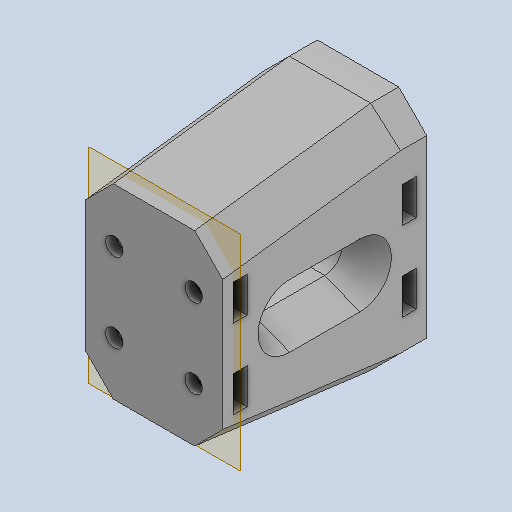
# Autodesk Inventor part: MCP-II
Saved by Autodesk Inventor 2026 (Build 300175050, 175E)
## iProperties
Created: 2025-12-08
Part Number: MCP-II
Material: Genérico
Document SubType Name: Modeling
Designer: user
Density: 1 g/cm^3
Appearance: Gris claro
Author: user
Autodesk Inventor part; units mm, degrees
ref_plane "YZ Plane" through (0, 0, 0) normal (1, 0, 0) x (0, 1, 0)
ref_plane "XZ Plane" through (0, 0, 0) normal (0, 1, 0) x (-1, 0, 0)
ref_plane "XY Plane" through (0, 0, 0) normal (0, 0, 1) x (1, 0, 0)
sketch "Boceto1" plane through (0, 0, 0) normal (0, 0, 1) x (1, 0, 0)
  line L0 (-9.8, -13.3) -> (-9.8, 13.3) projected
  line L1 (9.8, 13.3) -> (-9.8, 13.3) projected
  line L2 (9.8, 13.3) -> (9.8, -13.3) projected
  line L3 (-9.8, -13.3) -> (9.8, -13.3) projected
  circle A0 centre (-8, -8) radius 0.8 projected
  circle A1 centre (8, 8) radius 0.8 projected
  circle A2 centre (-8, 8) radius 0.8 projected
  circle A3 centre (0, 0) radius 4 projected
  circle A4 centre (0, -6) radius 1.025 projected
  circle A5 centre (-6, 0) radius 1.025 projected
  circle A6 centre (0, 6) radius 1.025 projected
  circle A7 centre (6, 0) radius 1.025 projected
  circle A8 centre (-5.6569, -5.6569) radius 1.025 projected
  circle A9 centre (-5.6569, 5.6569) radius 1.025 projected
  circle A10 centre (5.6569, 5.6569) radius 1.025 projected
  circle A11 centre (5.6569, -5.6569) radius 1.025 projected
  circle A12 centre (3, -9) radius 1.025 projected
  circle A13 centre (-3, -9) radius 1.025 projected
  circle A14 centre (3, 9) radius 1.025 projected
  circle A15 centre (-3, 9) radius 1.025 projected
  circle A16 centre (8, -8) radius 0.8 projected
  circle A17 centre (5.6569, 5.6569) radius 1.25
  circle A18 centre (5.6569, -5.6569) radius 1.25
  circle A19 centre (-5.6569, -5.6569) radius 1.25
  circle A20 centre (-5.6569, 5.6569) radius 1.25
  line L4 (9.7, -16.5) -> (-9.7, -16.5) projected
  line L5 (9.7, 16.5) -> (-9.7, 16.5) projected
  line L6 (9.8, -13.3) -> (-9.8, -13.3)
  line L7 (-9.8, -13.3) -> (-9.8, -16.5)
  line L8 (-9.8, -16.5) -> (9.8, -16.5)
  line L9 (9.8, -16.5) -> (9.8, -13.3)
  line L10 (9.8, 13.3) -> (-9.8, 13.3)
  line L11 (-9.8, 13.3) -> (-9.8, 16.5)
  line L12 (-9.8, 16.5) -> (9.8, 16.5)
  line L13 (9.8, 16.5) -> (9.8, 13.3)
  point P0 (0, 0)
  dimension "d30" = 2.5
  constraints: 16 end point, 4 centre point, 4 parallel, 3 equal radius, 2 collinear, 2 horizontal, 2 perpendicular, 2 point on line
  measures "d30" diameter of A17
extrude "Extrusión1" add sketch "Boceto1" along normal blind 14.5465 contours L0 L1 L2 L3 | L3 L9 L8 L4 L7 | L11 L12 L5 L13 L1 | A0 | A1 | A2 | A3 | A4 | A5 | A6 | A7 | A12 | A13 | A14 | A15 | A16
ref_plane "Plano de trabajo1" through (0, 0, 13.0465) normal (0, 0, 1) x (-1, 0, 0)
sketch "Boceto2" plane through (0, 0, 13.0465) normal (0, 0, 1) x (-1, 0, 0)
  arc A0 (1.1547, -3.8297) -> (-1.1547, -3.8297) centre (0, 0) ccw construction
  line L0 (-1.1547, -3.8297) -> (-1.1547, -4) construction
  line L1 (-1.1547, -4) -> (-1.6071, -4.7835) construction
  line L2 (-1.6071, -4.7835) -> (-1.5031, -4.8435) construction
  line L3 (-1.5031, -4.8435) -> (-1.7531, -5.2765) construction
  line L4 (-1.7531, -5.2765) -> (-1.8571, -5.2165) construction
  line L5 (-1.8571, -5.2165) -> (-2.3094, -6) construction
  line L6 (-2.3094, -6) -> (-1.9919, -6.55) construction
  arc A1 (-2.2517, -7) -> (-1.9919, -6.55) centre (-2.2517, -6.7) ccw construction
  line L7 (-2.2517, -7) -> (-2.75, -7) construction
  line L8 (-2.75, -7) -> (-2.75, -7.12) construction
  line L9 (-2.75, -7.12) -> (-3.25, -7.12) construction
  line L10 (-3.25, -7.12) -> (-3.25, -7) construction
  line L11 (-3.25, -7) -> (-4.1547, -7) construction
  line L12 (-4.1547, -7) -> (-4.3224, -6.789) construction
  arc A2 (-4.3224, -6.789) -> (-4.8553, -7.2125) centre (-5.6569, -5.6569) ccw construction
  line L13 (-4.8553, -7.2125) -> (-4.5206, -7.6337) construction
  line L14 (-4.5206, -7.6337) -> (-5.3094, -9) construction
  line L15 (-5.3094, -9) -> (-4.8571, -9.7835) construction
  line L16 (-4.8571, -9.7835) -> (-4.7531, -9.7235) construction
  line L17 (-4.7531, -9.7235) -> (-4.5031, -10.1565) construction
  line L18 (-4.5031, -10.1565) -> (-4.6071, -10.2165) construction
  line L19 (-4.6071, -10.2165) -> (-4.1547, -11) construction
  line L20 (-4.1547, -11) -> (-1.8453, -11) construction
  line L21 (-1.8453, -11) -> (-1.3929, -10.2165) construction
  line L22 (-1.3929, -10.2165) -> (-1.4969, -10.1565) construction
  line L23 (-1.4969, -10.1565) -> (-1.2469, -9.7235) construction
  line L24 (-1.2469, -9.7235) -> (-1.1429, -9.7835) construction
  line L25 (-1.1429, -9.7835) -> (-0.6906, -9) construction
  line L26 (-0.6906, -9) -> (-1.0081, -8.45) construction
  arc A3 (-0.7483, -8) -> (-1.0081, -8.45) centre (-0.7483, -8.3) ccw construction
  line L27 (-0.7483, -8) -> (-0.25, -8) construction
  line L28 (-0.25, -8) -> (-0.25, -7.88) construction
  line L29 (-0.25, -7.88) -> (0.25, -7.88) construction
  line L30 (0.25, -7.88) -> (0.25, -8) construction
  line L31 (0.25, -8) -> (0.7483, -8) construction
  arc A4 (1.0081, -8.45) -> (0.7483, -8) centre (0.7483, -8.3) ccw construction
  line L32 (1.0081, -8.45) -> (0.6906, -9) construction
  line L33 (0.6906, -9) -> (1.1429, -9.7835) construction
  line L34 (1.1429, -9.7835) -> (1.2469, -9.7235) construction
  line L35 (1.2469, -9.7235) -> (1.4969, -10.1565) construction
  line L36 (1.4969, -10.1565) -> (1.3929, -10.2165) construction
  line L37 (1.3929, -10.2165) -> (1.8453, -11) construction
  line L38 (1.8453, -11) -> (4.1547, -11) construction
  line L39 (4.1547, -11) -> (4.6071, -10.2165) construction
  line L40 (4.6071, -10.2165) -> (4.5031, -10.1565) construction
  line L41 (4.5031, -10.1565) -> (4.7531, -9.7235) construction
  line L42 (4.7531, -9.7235) -> (4.8571, -9.7835) construction
  line L43 (4.8571, -9.7835) -> (5.3094, -9) construction
  line L44 (5.3094, -9) -> (4.5206, -7.6337) construction
  line L45 (4.5206, -7.6337) -> (4.8553, -7.2125) construction
  arc A5 (4.8553, -7.2125) -> (4.3224, -6.789) centre (5.6569, -5.6569) ccw construction
  line L46 (4.3224, -6.789) -> (4.1547, -7) construction
  line L47 (4.1547, -7) -> (3.25, -7) construction
  line L48 (3.25, -7) -> (3.25, -7.12) construction
  line L49 (3.25, -7.12) -> (2.75, -7.12) construction
  line L50 (2.75, -7.12) -> (2.75, -7) construction
  line L51 (2.75, -7) -> (2.2517, -7) construction
  arc A6 (1.9919, -6.55) -> (2.2517, -7) centre (2.2517, -6.7) ccw construction
  line L52 (1.9919, -6.55) -> (2.3094, -6) construction
  line L53 (2.3094, -6) -> (1.8571, -5.2165) construction
  line L54 (1.8571, -5.2165) -> (1.7531, -5.2765) construction
  line L55 (1.7531, -5.2765) -> (1.5031, -4.8435) construction
  line L56 (1.5031, -4.8435) -> (1.6071, -4.7835) construction
  line L57 (1.6071, -4.7835) -> (1.1547, -4) construction
  line L58 (1.1547, -4) -> (1.1547, -3.8297) construction
  circle A7 centre (0, -6) radius 1.025 construction
  circle A8 centre (5.6569, -5.6569) radius 1.025 construction
  circle A9 centre (-5.6569, -5.6569) radius 1.025 construction
  circle A10 centre (-3, -9) radius 1.025 construction
  circle A11 centre (3, -9) radius 1.025 construction
  line L59 (7.6569, 6.8116) -> (7.6569, 4.5022) construction
  line L60 (7.6569, 4.5022) -> (5.6569, 3.3475) construction
  line L61 (5.6569, 3.3475) -> (3.6569, 4.5022) construction
  line L62 (3.6569, 4.5022) -> (3.6569, 6.8116) construction
  line L63 (3.6569, 6.8116) -> (5.6569, 7.9663) construction
  line L64 (5.6569, 7.9663) -> (7.6569, 6.8116) construction
  arc A12 (1.1547, 3.8297) -> (-1.1547, 3.8297) centre (0, 0) ccw construction
  line L65 (1.1547, 3.8297) -> (1.1547, 4) construction
  line L66 (1.1547, 4) -> (1.6071, 4.7835) construction
  line L67 (1.6071, 4.7835) -> (1.5031, 4.8435) construction
  line L68 (1.5031, 4.8435) -> (1.7531, 5.2765) construction
  line L69 (1.7531, 5.2765) -> (1.8571, 5.2165) construction
  line L70 (1.8571, 5.2165) -> (2.3094, 6) construction
  line L71 (2.3094, 6) -> (1.9919, 6.55) construction
  arc A13 (2.2517, 7) -> (1.9919, 6.55) centre (2.2517, 6.7) ccw construction
  line L72 (2.2517, 7) -> (2.75, 7) construction
  line L73 (2.75, 7) -> (2.75, 7.12) construction
  line L74 (2.75, 7.12) -> (3.25, 7.12) construction
  line L75 (3.25, 7.12) -> (3.25, 7) construction
  line L76 (3.25, 7) -> (4.1547, 7) construction
  line L77 (4.1547, 7) -> (4.3224, 6.789) construction
  arc A14 (4.3224, 6.789) -> (4.8553, 7.2125) centre (5.6569, 5.6569) ccw construction
  line L78 (4.8553, 7.2125) -> (4.5206, 7.6337) construction
  line L79 (4.5206, 7.6337) -> (5.3094, 9) construction
  line L80 (5.3094, 9) -> (4.8571, 9.7835) construction
  line L81 (4.8571, 9.7835) -> (4.7531, 9.7235) construction
  line L82 (4.7531, 9.7235) -> (4.5031, 10.1565) construction
  line L83 (4.5031, 10.1565) -> (4.6071, 10.2165) construction
  line L84 (4.6071, 10.2165) -> (4.1547, 11) construction
  line L85 (4.1547, 11) -> (1.8453, 11) construction
  line L86 (1.8453, 11) -> (1.3929, 10.2165) construction
  line L87 (1.3929, 10.2165) -> (1.4969, 10.1565) construction
  line L88 (1.4969, 10.1565) -> (1.2469, 9.7235) construction
  line L89 (1.2469, 9.7235) -> (1.1429, 9.7835) construction
  line L90 (1.1429, 9.7835) -> (0.6906, 9) construction
  line L91 (0.6906, 9) -> (1.0081, 8.45) construction
  arc A15 (0.7483, 8) -> (1.0081, 8.45) centre (0.7483, 8.3) ccw construction
  line L92 (0.7483, 8) -> (0.25, 8) construction
  line L93 (0.25, 8) -> (0.25, 7.88) construction
  line L94 (0.25, 7.88) -> (-0.25, 7.88) construction
  line L95 (-0.25, 7.88) -> (-0.25, 8) construction
  line L96 (-0.25, 8) -> (-0.7483, 8) construction
  arc A16 (-1.0081, 8.45) -> (-0.7483, 8) centre (-0.7483, 8.3) ccw construction
  line L97 (-1.0081, 8.45) -> (-0.6906, 9) construction
  line L98 (-0.6906, 9) -> (-1.1429, 9.7835) construction
  line L99 (-1.1429, 9.7835) -> (-1.2469, 9.7235) construction
  line L100 (-1.2469, 9.7235) -> (-1.4969, 10.1565) construction
  line L101 (-1.4969, 10.1565) -> (-1.3929, 10.2165) construction
  line L102 (-1.3929, 10.2165) -> (-1.8453, 11) construction
  line L103 (-1.8453, 11) -> (-4.1547, 11) construction
  line L104 (-4.1547, 11) -> (-4.6071, 10.2165) construction
  line L105 (-4.6071, 10.2165) -> (-4.5031, 10.1565) construction
  line L106 (-4.5031, 10.1565) -> (-4.7531, 9.7235) construction
  line L107 (-4.7531, 9.7235) -> (-4.8571, 9.7835) construction
  line L108 (-4.8571, 9.7835) -> (-5.3094, 9) construction
  line L109 (-5.3094, 9) -> (-4.5206, 7.6337) construction
  line L110 (-4.5206, 7.6337) -> (-4.8553, 7.2125) construction
  arc A17 (-4.8553, 7.2125) -> (-4.3224, 6.789) centre (-5.6569, 5.6569) ccw construction
  line L111 (-4.3224, 6.789) -> (-4.1547, 7) construction
  line L112 (-4.1547, 7) -> (-3.25, 7) construction
  line L113 (-3.25, 7) -> (-3.25, 7.12) construction
  line L114 (-3.25, 7.12) -> (-2.75, 7.12) construction
  line L115 (-2.75, 7.12) -> (-2.75, 7) construction
  line L116 (-2.75, 7) -> (-2.2517, 7) construction
  arc A18 (-1.9919, 6.55) -> (-2.2517, 7) centre (-2.2517, 6.7) ccw construction
  line L117 (-1.9919, 6.55) -> (-2.3094, 6) construction
  line L118 (-2.3094, 6) -> (-1.8571, 5.2165) construction
  line L119 (-1.8571, 5.2165) -> (-1.7531, 5.2765) construction
  line L120 (-1.7531, 5.2765) -> (-1.5031, 4.8435) construction
  line L121 (-1.5031, 4.8435) -> (-1.6071, 4.7835) construction
  line L122 (-1.6071, 4.7835) -> (-1.1547, 4) construction
  line L123 (-1.1547, 4) -> (-1.1547, 3.8297) construction
  circle A19 centre (0, 6) radius 1.025 construction
  circle A20 centre (5.6569, 5.6569) radius 1.025 construction
  circle A21 centre (-5.6569, 5.6569) radius 1.025 construction
  circle A22 centre (-3, 9) radius 1.025 construction
  circle A23 centre (3, 9) radius 1.025 construction
  line L124 (7.8569, 6.927) -> (7.8569, 4.3867)
  line L125 (7.8569, 4.3867) -> (5.6569, 3.1165)
  line L126 (5.6569, 3.1165) -> (3.4569, 4.3867)
  line L127 (3.4569, 4.3867) -> (3.4569, 6.927)
  line L128 (3.4569, 6.927) -> (5.6569, 8.1972)
  line L129 (5.6569, 8.1972) -> (7.8569, 6.927)
  circle A24 centre (-5.6569, -5.6569) radius 1.25 projected
  circle A25 centre (-5.6569, 5.6569) radius 1.25 projected
  circle A26 centre (5.6569, 5.6569) radius 1.25 projected
  circle A27 centre (5.6569, -5.6569) radius 1.25 projected
  line L130 (5.6569, 3.1165) -> (9.8, 3.1165)
  line L131 (5.6569, 8.1972) -> (9.8, 8.1972)
  line L132 (-9.5516, 0) -> (9.5516, 0) construction
  line L133 (0, -13.1978) -> (0, 13.1978) construction
  line L134 (7.8569, -6.927) -> (7.8569, -4.3867)
  line L135 (7.8569, -4.3867) -> (5.6569, -3.1165)
  line L136 (5.6569, -3.1165) -> (3.4569, -4.3867)
  line L137 (3.4569, -4.3867) -> (3.4569, -6.927)
  line L138 (3.4569, -6.927) -> (5.6569, -8.1972)
  line L139 (5.6569, -8.1972) -> (7.8569, -6.927)
  line L140 (5.6569, -3.1165) -> (9.8, -3.1165)
  line L141 (5.6569, -8.1972) -> (9.8, -8.1972)
  line L142 (-7.8569, 6.927) -> (-7.8569, 4.3867)
  line L143 (-7.8569, 4.3867) -> (-5.6569, 3.1165)
  line L144 (-5.6569, 3.1165) -> (-3.4569, 4.3867)
  line L145 (-3.4569, 4.3867) -> (-3.4569, 6.927)
  line L146 (-3.4569, 6.927) -> (-5.6569, 8.1972)
  line L147 (-5.6569, 8.1972) -> (-7.8569, 6.927)
  line L148 (-5.6569, 3.1165) -> (-9.8, 3.1165)
  line L149 (-5.6569, 8.1972) -> (-9.8, 8.1972)
  line L150 (-5.6569, -3.1165) -> (-9.8, -3.1165)
  line L151 (-5.6569, -3.1165) -> (-3.4569, -4.3867)
  line L152 (-3.4569, -4.3867) -> (-3.4569, -6.927)
  line L153 (-3.4569, -6.927) -> (-5.6569, -8.1972)
  line L154 (-5.6569, -8.1972) -> (-9.8, -8.1972)
  line L155 (-5.6569, -8.1972) -> (-7.8569, -6.927)
  line L156 (-7.8569, -6.927) -> (-7.8569, -4.3867)
  line L157 (-7.8569, -4.3867) -> (-5.6569, -3.1165)
  line L158 (-9.8, 16.5) -> (9.8, 16.5) projected
  line L159 (9.8, 16.5) -> (9.8, -16.5) projected
  line L160 (9.8, -16.5) -> (-9.8, -16.5) projected
  line L161 (-9.8, -16.5) -> (-9.8, 16.5) projected
  point P0 (0, 0)
  point P1 (0, 0)
  point P2 (0, 0)
  dimension "d3" = 4.6188
  dimension "d101" = 0.2
  constraints: 80 end point, 24 symmetric about line, 4 midpoint, 2 coincident, 2 vertical, 1 horizontal, 18 other
  measures "d3" distance of L59.end L62.end
  measures "d101" distance between parallel lines of L64 L129
extrude "Extrusión2" cut sketch "Boceto2" against normal blind 2 contours L129 L131 L159 L130 L125 L124 | L124 L125 L126 L127 L128 L129 | L159 L141 L139 L134 L135 L140 | L135 L134 L139 L138 L137 L136 | L149 L147 L142 L143 L148 L161 | L146 L145 L144 L143 L142 L147 | L150 L157 L156 L155 L154 L161 | L151 L152 L153 L155 L156 L157 | A24 | A25 | A26 | A27
mirror "Simetría2" about plane through (0, 0, 0) normal (0, 0, 1)
sketch "Boceto4" plane through (0, 0, 14.5465) normal (0, 0, 1) x (1, 0, 0)
  circle A0 centre (-5.6569, -5.6569) radius 1.25 construction
  circle A1 centre (5.6569, 5.6569) radius 1.25 construction
  circle A2 centre (-5.6569, -5.6569) radius 2.3094 construction
  circle A3 centre (-5.6569, -5.6569) radius 3.1431
  circle A4 centre (5.6569, 5.6569) radius 3.1431
  point P0 (0, 0)
  point P1 (-5.6569, -7.9663)
  point P2 (-7.6569, -4.5022)
  point P3 (-3.6569, -4.5022)
  dimension "d84" = 360
  constraints: 3 centre point, 3 point on circle, 5 other
extrude "Extrusión3" [suppressed]
chamfer "Chaflán1" [suppressed]
chamfer "Chaflán4" [suppressed]
pattern_circular "Patrón circular1" [suppressed]
chamfer "Chaflán7" distance 3.2 distance2 25.093 2 edges at (0, -16.5, 14.5465) (0, 16.5, 14.5465) measured on face at (-1.6489, -13.2285, 14.5465)
chamfer "Chaflán2" distance 4 angle 45 8 edges at (-9.8, -14.9, 2) (9.8, -14.9, 2) (9.8, 14.9, 2) (-9.8, 14.9, 2) (9.8, -16.5, -12.5465) (-9.8, -16.5, -12.5465) (9.8, 16.5, -12.5465) (-9.8, 16.5, -12.5465)
sketch "Boceto5" plane through (0, 0, 0) normal (1, 0, 0) x (0, 1, 0)
  line L0 (13.3, -14.5465) -> (-13.3, -14.5465) construction
  line L1 (0, -5) -> (0, 5) construction
  line L2 (2.5, -5) -> (2.5, 5)
  line L3 (-2.5, 5) -> (-2.5, -5)
  arc A0 (-2.5, -5) -> (2.5, -5) centre (0, -5) ccw
  arc A1 (2.5, 5) -> (-2.5, 5) centre (0, 5) ccw
  line L4 (10.1, 14.5465) -> (-10.1, 14.5465) projected
  line L5 (10.1, 14.5465) -> (13.3, -14.5465) projected
  line L6 (-13.3, -14.5465) -> (-10.1, 14.5465) projected
  point P0 (0, 0)
  dimension "d91" = 5
  dimension "d104" = 15
  constraints: 8 end point, 4 point on circle, 4 tangent, 2 centre point, 1 midpoint, 1 parallel, 1 vertical
  measures "d91" diameter of A1
extrude "Extrusión4" cut sketch "Boceto5" along normal through all both and the other way through all
chamfer "Chaflán5" distance 2 distance2 5 4 edges at (9.8, -2.5, 0) (9.8, 0, 7.5) (9.8, 2.5, 0) (9.8, 0, -7.5) measured on face at (9.8, -7.7324, 1.7487)
chamfer "Chaflán6" distance 2 distance2 5 4 edges at (-9.8, 0, -7.5) (-9.8, 2.5, 0) (-9.8, 0, 7.5) (-9.8, -2.5, 0) measured on face at (-9.8, -7.7324, 1.7487)
equation "\"d3\" = d2"
equation "\"d2\" = 4.618802"
